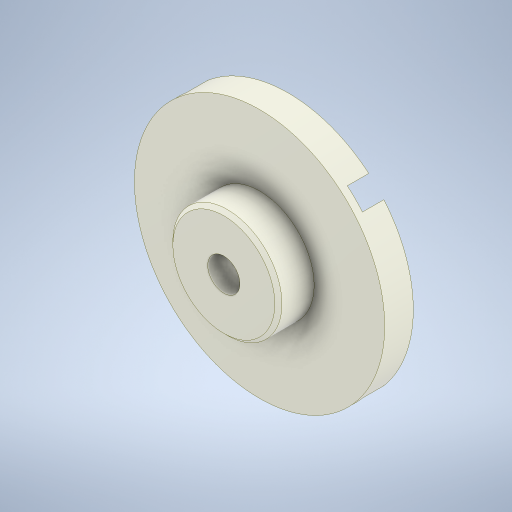
# Autodesk Inventor part: chuck_v03_1.5inset
Saved by Autodesk Inventor 2023.1 (Build 271208000, 208)
## iProperties
Created: 2019-07-31
Part Number: chuck_v03_1.5inset
Material: Polytetrafluoroethylene
Document SubType Name: Modeling
Designer: Timo
Density: 2.02 g/cm^3
Appearance: Smooth - Ivory
Author: Timo
Autodesk Inventor part; units mm, degrees
ref_plane "XZ Plane" through (0, 0, 0) normal (0, 1, 0) x (-1, 0, 0)
ref_plane "XY Plane" through (0, 0, 0) normal (0, 0, 1) x (1, 0, 0)
sketch "Sketch1" plane through (0, 0, 0) normal (0, 0, 1) x (1, 0, 0)
  circle A0 centre (0, 0) radius 17.5
  dimension "d0" = 35
  constraints: 1 centre point, 1 coincident
  measures "d0" diameter of A0
extrude "Extrusion1" add sketch "Sketch1" along normal blind 4
sketch "Sketch2" plane through (0, 0, 4) normal (0, 0, 1) x (1, 0, 0)
  circle A0 centre (0, 0) radius 7.625
  dimension "d3" = 15.25
  constraints: 1 centre point, 1 coincident
  measures "d3" diameter of A0
extrude "Extrusion2" add sketch "Sketch2" along normal blind 5
chamfer "Chamfer1" distance 0.5 angle 45 1 edges at (-7.625, 0, 9)
sketch "Sketch3" plane through (0, 0, 0) normal (0, 0, -1) x (-1, 0, 0)
  line L0 (-7.4, -7.4) -> (7.4, -7.4)
  line L1 (7.4, -7.4) -> (7.4, 7.4)
  line L2 (7.4, 7.4) -> (-7.4, 7.4)
  line L3 (-7.4, 7.4) -> (-7.4, -7.4)
  line L4 (-7.4, -7.4) -> (7.4, 7.4) construction
  line L5 (7.4, -7.4) -> (-7.4, 7.4) construction
  point P0 (0, 0)
  dimension "d15" = 1.5
  dimension "d9" = 14.8
  constraints: 12 end point, 2 midpoint, 2 parallel, 2 perpendicular, 1 horizontal
  measures "d9" distance of L1.end L2.end
extrude "Extrusion3" cut sketch "Sketch3" against normal blind 1.2
sketch "Sketch4" plane through (0, 0, 0) normal (0, 0, -1) x (-1, 0, 0)
  line L0 (-7.4, -7.4) -> (-7.4, 7.4) projected
  circle A0 centre (-7.4, 7.4) radius 3
  point P0 (0, 0)
  dimension "d12" = 6
  constraints: 1 centre point
  measures "d12" diameter of A0
extrude "Extrusion4" cut sketch "Sketch4" against normal blind 3
sketch "Sketch5" plane through (0, 0, 0) normal (0, 0, -1) x (-1, 0, 0)
  circle A0 centre (-7.4, 7.4) radius 3 projected
  line L0 (-7.4, 7.4) -> (-12.3744, 12.3744) construction
  circle A1 centre (0, 0) radius 17.5 projected
  line L1 (-6.3393, 8.4607) -> (-11.3137, 13.435)
  line L2 (-13.435, 11.3137) -> (-8.4607, 6.3393)
  arc A2 (-8.4607, 6.3393) -> (-6.3393, 8.4607) centre (-7.4, 7.4) ccw
  arc A3 (-11.3137, 13.435) -> (-13.435, 11.3137) centre (-12.3744, 12.3744) ccw
  line L3 (0, -24.5) -> (0, 24.5) projected
  point P0 (-9.8872, 9.8872)
  point P1 (-13.3895, 11.2682)
  point P2 (-10.2978, 8.1765)
  point P3 (-8.1765, 10.2978)
  point P4 (-11.2682, 13.3895)
  dimension "d15" = 1.5
  dimension "d16" = 45
  constraints: 8 end point, 4 point on circle, 4 tangent, 2 centre point, 1 midpoint, 1 parallel, 2 other
  measures "d15" radius of A3
  measures "d16" angle of L3 L0
extrude "Extrusion5" cut sketch "Sketch5" against normal up to surface (3 mm away) contours A0 L2 A1 L1
pattern_circular "Circular Pattern1" count 4 over 360 about axis through (0, 0, -10) along (0, 0, 1) of "Extrusion4", "Extrusion5"
sketch "Sketch6" plane through (0, 0, 1.2) normal (0, 0, -1) x (-1, 0, 0)
  circle A0 centre (0, 0) radius 2.25
  dimension "d22" = 4.5
  constraints: 1 centre point, 1 coincident
  measures "d22" diameter of A0
extrude "Extrusion6" cut sketch "Sketch6" against normal through all
ref_plane "Work Plane1" through (0, 0, 0) normal (0.7071, 0.7071, 0) x (0, 0, 1)
sketch "Sketch7" plane through (0, 0, 1.2) normal (0, 0, -1) x (-1, 0, 0)
  line L0 (7.4, 5.1639) -> (5.4, 5.1639)
  line L1 (5.4, 5.1639) -> (5.4, -5.1639)
  line L2 (5.4, -5.1639) -> (7.4, -5.1639)
  line L3 (7.4, -5.1639) -> (7.4, 5.1639)
  line L4 (7.4, 4.4) -> (7.4, -4.4) projected
  arc A0 (4.4, 7.4) -> (7.4, 4.4) centre (7.4, 7.4) ccw projected
  arc A1 (7.4, -4.4) -> (4.4, -7.4) centre (7.4, -7.4) ccw projected
  point P0 (0, 0)
  dimension "d26" = 2
  constraints: 8 end point, 2 parallel, 2 point on circle, 1 collinear, 1 horizontal, 1 perpendicular
  measures "d26" distance between parallel lines of L3 L1
extrude "Extrusion7" cut sketch "Sketch7" against normal up to surface (1.8 mm away)
pattern_circular "Circular Pattern2" count 4 over 360 about axis through (0, 0, -10) along (0, 0, 1) of "Extrusion7"
body "Solid1"
